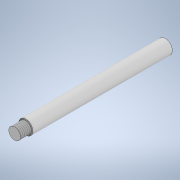
# Autodesk Inventor part: Eje roscado base soporte tubo
Saved by Autodesk Inventor 2021 (Build 250183000, 183)
## iProperties
Created: 2021-05-29
Part Number: Eje roscado base soporte tubo
Material: Generic
Document SubType Name: Modeling
Designer: Nelson
Density: 1 g/cm^3
Appearance: Default
Author: Nelson
Autodesk Inventor part; units mm, degrees
ref_plane "YZ Plane" through (0, 0, 0) normal (1, 0, 0) x (0, 1, 0)
ref_plane "XZ Plane" through (0, 0, 0) normal (0, 1, 0) x (-1, 0, 0)
ref_plane "XY Plane" through (0, 0, 0) normal (0, 0, 1) x (1, 0, 0)
sketch "Sketch2" plane through (0, 0, 0) normal (1, 0, 0) x (0, 1, 0)
  line L0 (0, 0) -> (7.9375, 0)
  line L1 (7.9375, 0) -> (7.9375, -15)
  line L2 (7.9375, -15) -> (9.525, -15)
  line L3 (0, -203.578) -> (0, 0)
  line L4 (9.525, -15) -> (9.525, -203.578)
  line L5 (9.525, -203.578) -> (0, -203.578)
  dimension "d7" = 7.9375
  dimension "d8" = 15
  dimension "d9" = 1.5875
  dimension "d23" = 188.578
  constraints: 12 end point, 3 horizontal, 2 vertical
  measures "d7" distance of L0.start L0.end
  measures "d8" distance of L0.end L1.end
  measures "d9" distance of L1.end L2.end
  measures "d23" distance of L2.end L4.end
revolve "Revolution1" add sketch "Sketch2" angle 360 about axis through (0, 0, -203.578) along (0, 0, 1)
thread "Thread4" size "5/8-11 UNC" class "2A" standard "ANSI Unified Screw Threads" full length
sketch "Sketch4" plane through (0, 0, -203.578) normal (0, 0, -1) x (-1, 0, 0)
  point P0 (0, 0)
  point P1 (0, 0)
  constraints: 1 coincident
hole "Hole1" at (0, 0, -203.578) direction (0, 0, 1) diameter 6.4008 depth 15 tip angle 137 thread size "5/16-18 UNC" class "2B" standard "ANSI Unified Screw Threads"
body "Solid2"
